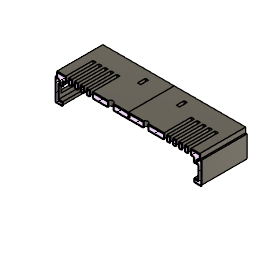
10.1 Screen Case Assembly (Autodesk Fusion 360 design; units mm, degrees)
part number: 2026-02-22-22-43-30-238
Autodesk Fusion 360 part; units mm, degrees
note: some values were not read from the file. Set by a fixed rule: which face or edge a step refers to.
(part 1 of 2)
sketch "Sketch1" plane through (0, 0, 0) normal (0, 0, 1) x (1, 0, 0)
  line L0 (117.5, -71.5) -> (-117.5, -71.5)
  line L1 (-117.5, -71.5) -> (-117.5, 71.5)
  line L2 (-117.5, 71.5) -> (117.5, 71.5)
  line L3 (117.5, 71.5) -> (117.5, -71.5)
  line L4 (117.5, -71.5) -> (-117.5, 71.5) construction
  line L5 (-117.5, -71.5) -> (117.5, 71.5) construction
  line L6 (-112.5, -66.5) -> (-112.5, 66.5)
  line L7 (-112.5, 66.5) -> (112.5, 66.5)
  line L8 (112.5, 66.5) -> (112.5, -66.5)
  line L9 (112.5, -66.5) -> (-112.5, -66.5)
  line L10 (122.5, -76.5) -> (-122.5, -76.5)
  line L11 (-122.5, -76.5) -> (-122.5, 76.5)
  line L12 (-122.5, 76.5) -> (122.5, 76.5)
  line L13 (122.5, 76.5) -> (122.5, -76.5)
  dimension "d1" = 235
  dimension "d2" = 143
  dimension "d3" = 5
  dimension "d4" = -5
  constraint horizontal L0
  constraint perpendicular L0 L1
  constraint parallel L0 L2
  constraint parallel L1 L3
  constraint coincident L4 origin
  constraint coincident L5 origin
  measures "d1" distance of L1.end L2.end
  measures "d2" distance of L0.end L1.end
extrude "Extrude1" add sketch "Sketch1" along normal blind 25 contours L0 L1 L2 L3 | L10 L11 L12 L13 makes body 1
ref_plane "WorkPlane1" through (0, 0, 12.5) normal (1, 0, 0) x (0, 1, 0)
sketch "Sketch2" plane through (0, 0, 0) normal (0, 0, -1) x (1, 0, 0)
  line L0 (112.5, 66.5) -> (112.5, -66.5)
  line L1 (112.5, -66.5) -> (-112.5, -66.5)
  line L2 (-112.5, -66.5) -> (-112.5, 66.5)
  line L3 (-112.5, 66.5) -> (112.5, 66.5)
  line L4 (-122.5, -76.5) -> (122.5, -76.5)
  line L5 (122.5, -76.5) -> (122.5, 76.5)
  line L6 (122.5, 76.5) -> (-122.5, 76.5)
  line L7 (-122.5, 76.5) -> (-122.5, -76.5)
sketch "Sketch3" plane through (0, 0, 25) normal (0, 0, 1) x (-1, 0, 0)
  line L0 (-112.5, -66.5) -> (-112.5, 66.5)
  line L1 (-112.5, 66.5) -> (112.5, 66.5)
  line L2 (112.5, 66.5) -> (112.5, -66.5)
  line L3 (112.5, -66.5) -> (-112.5, -66.5)
  line L4 (-122.5, -76.5) -> (122.5, -76.5)
  line L5 (122.5, -76.5) -> (122.5, 76.5)
  line L6 (122.5, 76.5) -> (-122.5, 76.5)
  line L7 (-122.5, 76.5) -> (-122.5, -76.5)
  line L8 (-112.5, 66.5) -> (112.5, 66.5)
  line L9 (-117.5, -71.5) -> (117.5, 71.5) construction
  line L10 (122.5, 76.5) -> (122.5, -76.5)
  line L11 (-112.5, -66.5) -> (-112.5, 66.5)
  line L12 (117.5, -71.5) -> (-117.5, 71.5) construction
  line L13 (117.5, -71.5) -> (-117.5, -71.5)
  line L14 (117.5, 71.5) -> (117.5, -71.5)
  line L15 (112.5, -66.5) -> (-112.5, -66.5)
  line L16 (-117.5, -71.5) -> (-117.5, 71.5)
  line L17 (-122.5, -76.5) -> (-122.5, 76.5)
  line L18 (112.5, 66.5) -> (112.5, -66.5)
  line L19 (-122.5, 76.5) -> (122.5, 76.5)
  line L20 (-117.5, 71.5) -> (117.5, 71.5)
  line L21 (122.5, -76.5) -> (-122.5, -76.5)
  dimension "d7" = 5
  dimension "d8" = -5
  dimension "d9" = 235
  dimension "d10" = 143
  constraint horizontal L13
  constraint perpendicular L13 L16
  constraint parallel L13 L20
  constraint parallel L14 L16
  constraint coincident origin L12
  constraint coincident origin L9
  measures "d9" distance of L12.end L9.end
  measures "d10" distance of L12.end L9.start
extrude "Extrude2" cut sketch "Sketch3" against normal blind 20 contours L13 L14 L16 L20 bodies 1
sketch "Sketch5" plane through (0, -71.5, 0) normal (0, 1, 0) x (-1, 0, 0)
  line L0 (117.5, 25) -> (-117.5, 25)
  line L1 (-117.5, 25) -> (-117.5, 5)
  line L2 (-117.5, 5) -> (117.5, 5)
  line L3 (117.5, 5) -> (117.5, 25)
sketch "Sketch6" plane through (0, 76.5, 0) normal (0, 1, 0) x (-1, 0, 0)
  line L0 (-122.5, 0) -> (122.5, 0)
  line L1 (122.5, 0) -> (122.5, 25)
  line L2 (122.5, 25) -> (-122.5, 25)
  line L3 (-122.5, 25) -> (-122.5, 0)
  line L4 (122.5, 25) -> (-122.5, 25)
  line L5 (-122.5, 25) -> (-122.5, 0)
  line L6 (-122.5, 0) -> (122.5, 0)
  line L7 (122.5, 0) -> (122.5, 25)
  line L8 (-117.5, 5) -> (117.5, 5)
  line L9 (117.5, 5) -> (117.5, 25)
  line L10 (117.5, 25) -> (-117.5, 25)
  line L11 (-117.5, 25) -> (-117.5, 5)
  line L12 (-117.5, 5) -> (-94.5, 5)
  line L13 (-94.5, 5) -> (-59, 5)
  line L14 (-59, 5) -> (-59, 12)
  line L15 (-59, 12) -> (-94.5, 12)
  line L16 (-94.5, 12) -> (-94.5, 5)
  dimension "d19" = 23
  dimension "d20" = 35.5
  dimension "d21" = 7
  constraint horizontal L4
  constraint vertical L5
  constraint horizontal L6
  constraint vertical L7
  constraint coincident L0.start L3.end
  constraint coincident L1.end L2.start
  constraint horizontal L8
  constraint vertical L9
  constraint horizontal L10
  constraint vertical L11
  constraint coincident L4 L9.end
  constraint horizontal L12
  constraint horizontal L13
  constraint vertical L14
  constraint horizontal L15
  constraint vertical L16
  measures "d19" distance of L8.start L12.end
  measures "d20" distance of L12.end L13.end
  measures "d21" distance of L12.end L15.end
extrude "Extrude3" cut sketch "Sketch6" against normal blind 8 contours L8 L13 L14 L15 L16 bodies 1
sketch "Sketch7" plane through (-117.5, 0, 0) normal (1, 0, 0) x (0, 1, 0)
  line L0 (71.5, 25) -> (-71.5, 25)
  line L1 (-71.5, 25) -> (-71.5, 5)
  line L2 (-71.5, 5) -> (71.5, 5)
  line L3 (71.5, 5) -> (71.5, 25)
  line L4 (71.5, 5) -> (44.8, 5)
  line L5 (50, 5) -> (14.4, 5)
  line L6 (14.4, 5) -> (14.4, 12)
  line L7 (14.4, 12) -> (50, 12)
  line L8 (50, 12) -> (50, 5)
  dimension "d24" = 26.7
  dimension "d25" = 35.6
  dimension "d26" = 7
  constraint coincident L2.end L3.start
  constraint perpendicular L3 L4
  constraint horizontal L5
  constraint vertical L6
  constraint horizontal L7
  constraint vertical L8
  constraint coincident L4 L5.start
  measures "d24" distance of L2.end L4.end
  measures "d25" distance of L5.start L5.end
  measures "d26" distance of L5.start L7.end
extrude "Extrude4" cut sketch "Sketch7" against normal blind 20 contours L2 L4 L5 L6 L7 L8 bodies 1
sketch "Sketch8" plane through (0, -76.5, 0) normal (0, -1, 0) x (1, 0, 0)
  line L0 (-122.5, 0) -> (122.5, 0)
  line L1 (122.5, 0) -> (122.5, 25)
  line L2 (122.5, 25) -> (-122.5, 25)
  line L3 (-122.5, 25) -> (-122.5, 0)
  line L4 (0, 0) -> (0, 30)
  constraint coincident L4.start origin
  constraint perpendicular L0 L4
sketch "Sketch9" plane through (0, 71.5, 0) normal (0, -1, 0) x (1, 0, 0)
  line L0 (117.5, 25) -> (-117.5, 25)
  line L1 (-117.5, 25) -> (-117.5, 5)
  line L2 (94.5, 5) -> (117.5, 5)
  line L3 (-117.5, 25) -> (117.5, 25)
  line L4 (117.5, 25) -> (117.5, 5)
  line L5 (117.5, 5) -> (-117.5, 5)
  line L6 (-117.5, 5) -> (-117.5, 25)
  line L7 (-117.5, 10.0628) -> (117.5, 10.0628)
  line L8 (117.5, 10.0628) -> (117.5, 15)
  line L9 (117.5, 15) -> (-117.5, 15)
  line L10 (-117.5, 15) -> (-117.5, 10.0628)
  line L11 (59, 5) -> (59, 12)
  line L12 (59, 12) -> (94.5, 12)
  line L13 (94.5, 12) -> (94.5, 5)
  line L14 (117.5, 5) -> (117.5, 25)
  line L15 (-117.5, 5) -> (59, 5)
  constraint horizontal L3
  constraint vertical L4
  constraint horizontal L5
  constraint vertical L6
  constraint coincident L2.end L4.end
  constraint coincident L0.end L1.start
  constraint horizontal L7
  constraint vertical L8
  constraint horizontal L9
  constraint vertical L10
  constraint midpoint L4 L8.end
  constraint coincident L6 L7.start
sketch "Sketch10" plane through (0, 0, 5) normal (0, 0, 1) x (-1, 0, 0)
  line L0 (-59, -71.5) -> (117.5, -71.5)
  line L1 (117.5, -71.5) -> (117.5, -50)
  line L2 (117.5, -50) -> (122.5, -50)
  line L3 (122.5, -50) -> (122.5, -14.4)
  line L4 (122.5, -14.4) -> (117.5, -14.4)
  line L5 (117.5, -14.4) -> (117.5, 71.5)
  line L6 (117.5, 71.5) -> (-117.5, 71.5)
  line L7 (-117.5, 71.5) -> (-117.5, -71.5)
  line L8 (-117.5, -71.5) -> (-94.5, -71.5)
  line L9 (-94.5, -71.5) -> (-94.5, -76.5)
  line L10 (-94.5, -76.5) -> (-59, -76.5)
  line L11 (-59, -76.5) -> (-59, -71.5)
  line L12 (-112.5, 66.5) -> (112.5, 66.5)
  line L13 (112.5, 66.5) -> (112.5, -66.5)
  line L14 (112.5, -66.5) -> (-112.5, -66.5)
  line L15 (-112.5, -66.5) -> (-112.5, 66.5)
  line L16 (117.5, -14.4) -> (122.5, -14.4)
  line L17 (122.5, -14.4) -> (122.5, -50)
  line L18 (122.5, -50) -> (117.5, -50)
  line L19 (117.5, -50) -> (117.5, -14.4)
  line L20 (117.5, -32.2) -> (122.5, -32.2)
  line L21 (120, -14.4) -> (120, -32.2)
  line L22 (120.4, -23.4) -> (119.6, -23.4)
  line L23 (119.6, -23.4) -> (119.6, -22.6)
  line L24 (119.6, -22.6) -> (120.4, -22.6)
  line L25 (120.4, -22.6) -> (120.4, -23.4)
  line L26 (120.4, -23.4) -> (119.6, -22.6) construction
  line L27 (119.6, -23.4) -> (120.4, -22.6) construction
  line L28 (120.4, -27.6) -> (119.6, -27.6)
  line L29 (119.6, -27.6) -> (119.6, -28.4)
  line L30 (119.6, -28.4) -> (120.4, -28.4)
  line L31 (120.4, -28.4) -> (120.4, -27.6)
  line L32 (120.4, -27.6) -> (119.6, -28.4) construction
  line L33 (119.6, -27.6) -> (120.4, -28.4) construction
  line L34 (120.4, -36) -> (120.4, -36.8)
  line L35 (120.4, -36.8) -> (119.6, -36.8)
  line L36 (119.6, -36.8) -> (119.6, -36)
  line L37 (119.6, -36) -> (120.4, -36)
  line L38 (120.4, -41.8) -> (120.4, -41)
  line L39 (119.6, -41.8) -> (120.4, -41.8)
  line L40 (120.4, -41) -> (119.6, -41)
  line L41 (119.6, -41) -> (119.6, -41.8)
  line L42 (120.4, -17.6) -> (119.6, -17.6)
  line L43 (119.6, -17.6) -> (119.6, -18.4)
  line L44 (119.6, -18.4) -> (120.4, -18.4)
  line L45 (120.4, -18.4) -> (120.4, -17.6)
  line L46 (120.4, -17.6) -> (119.6, -18.4) construction
  line L47 (119.6, -17.6) -> (120.4, -18.4) construction
  line L48 (119.6, -46.8) -> (119.6, -46)
  line L49 (120.4, -46.8) -> (119.6, -46.8)
  line L50 (120.4, -46) -> (120.4, -46.8)
  line L51 (119.6, -46) -> (120.4, -46)
  line L52 (119.6, -31.8) -> (120.4, -31.8)
  line L53 (120.4, -31.8) -> (120.4, -32.6)
  line L54 (120.4, -32.6) -> (119.6, -32.6)
  line L55 (119.6, -32.6) -> (119.6, -31.8)
  line L56 (119.6, -31.8) -> (120.4, -32.6) construction
  line L57 (120.4, -31.8) -> (119.6, -32.6) construction
  point P0 (120, -23)
  point P1 (120, -28)
  point P2 (120, -18)
  point P3 (120, -46.4)
  point P4 (120, -32.2)
  dimension "d32" = 0.8
  dimension "d33" = 0.8
  dimension "d34" = 0.8
  dimension "d35" = 0.8
  dimension "d38" = 0.8
  dimension "d39" = 0.8
  dimension "d56" = 0.8
  dimension "d57" = 0.8
  constraint horizontal L16
  constraint vertical L17
  constraint horizontal L18
  constraint vertical L19
  constraint coincident L2.end L3.start
  constraint coincident L4.end L5.start
  constraint midpoint L19 L20.start
  constraint midpoint L3 L20.end
  constraint midpoint L4 L21.start
  constraint midpoint L20 P4
  constraint horizontal L22
  constraint perpendicular L22 L23
  constraint parallel L22 L24
  constraint parallel L23 L25
  constraint coincident L26 P0
  constraint coincident L27 P0
  constraint coincident L21 P0
  constraint horizontal L28
  constraint perpendicular L28 L29
  constraint parallel L28 L30
  constraint parallel L29 L31
  constraint coincident L32 P1
  constraint coincident L33 P1
  constraint coincident L21 P1
  constraint symmetric L20 L22.start L38.end
  constraint symmetric L20 L22.end L40.end
  constraint symmetric L20 L23.end L39.start
  constraint symmetric L20 L24.end L38.start
  constraint symmetric L20 L28.start L34.end
  constraint symmetric L20 L28.end L35.end
  constraint symmetric L20 L29.end L36.end
  constraint symmetric L20 L30.end L34.start
  constraint horizontal L42
  constraint perpendicular L42 L43
  constraint parallel L42 L44
  constraint parallel L43 L45
  constraint coincident L46 P2
  constraint coincident L47 P2
  constraint coincident L21 P2
  constraint symmetric L20 L42.start L49.start
  constraint symmetric L20 L42.end L48.start
  constraint symmetric L20 L43.end L48.end
  constraint symmetric L20 L44.end L50.start
  constraint symmetric L20 P2 P3
  constraint horizontal L52
  constraint perpendicular L52 L53
  constraint parallel L52 L54
  constraint parallel L53 L55
  constraint coincident L56 P4
  constraint coincident L57 P4
  constraint coincident P4 L21.end
  measures "d32" distance of L23.end L24.end
  measures "d33" distance of L22.end L23.end
  measures "d34" distance of L29.end L30.end
  measures "d35" distance of L28.end L29.end
  measures "d38" distance of L43.end L44.end
  measures "d39" distance of L42.end L43.end
  measures "d56" distance of L53.end L54.end
  measures "d57" distance of L52.end L53.end
sketch "Sketch11" plane through (0, 0, 5) normal (0, 0, 1) x (-1, 0, 0)
  line L0 (-59, -71.5) -> (117.5, -71.5)
  line L1 (117.5, -71.5) -> (117.5, -50)
  line L2 (117.5, -50) -> (122.5, -50)
  line L3 (122.5, -50) -> (122.5, -14.4)
  line L4 (122.5, -14.4) -> (117.5, -14.4)
  line L5 (117.5, -14.4) -> (117.5, 71.5)
  line L6 (117.5, 71.5) -> (-117.5, 71.5)
  line L7 (-117.5, 71.5) -> (-117.5, -71.5)
  line L8 (-117.5, -71.5) -> (-94.5, -71.5)
  line L9 (-94.5, -71.5) -> (-94.5, -76.5)
  line L10 (-94.5, -76.5) -> (-59, -76.5)
  line L11 (-59, -76.5) -> (-59, -71.5)
  line L12 (-112.5, 66.5) -> (112.5, 66.5)
  line L13 (112.5, 66.5) -> (112.5, -66.5)
  line L14 (112.5, -66.5) -> (-112.5, -66.5)
  line L15 (-112.5, -66.5) -> (-112.5, 66.5)
  line L16 (-59, -76.5) -> (-94.5, -76.5)
  line L17 (-94.5, -76.5) -> (-94.5, -71.5)
  line L18 (-94.5, -71.5) -> (-59, -71.5)
  line L19 (-59, -71.5) -> (-59, -76.5)
  line L20 (-77.15, -73.6) -> (-76.35, -73.6)
  line L21 (-76.35, -73.6) -> (-76.35, -74.4)
  line L22 (-76.35, -74.4) -> (-77.15, -74.4)
  line L23 (-77.15, -74.4) -> (-77.15, -73.6)
  line L24 (-77.15, -73.6) -> (-76.35, -74.4) construction
  line L25 (-76.35, -73.6) -> (-77.15, -74.4) construction
  line L26 (-61.4, -73.6) -> (-60.6, -73.6)
  line L27 (-60.6, -73.6) -> (-60.6, -74.4)
  line L28 (-60.6, -74.4) -> (-61.4, -74.4)
  line L29 (-61.4, -74.4) -> (-61.4, -73.6)
  line L30 (-61.4, -73.6) -> (-60.6, -74.4) construction
  line L31 (-60.6, -73.6) -> (-61.4, -74.4) construction
  line L32 (-64.4, -73.6) -> (-63.6, -73.6)
  line L33 (-63.6, -73.6) -> (-63.6, -74.4)
  line L34 (-63.6, -74.4) -> (-64.4, -74.4)
  line L35 (-64.4, -74.4) -> (-64.4, -73.6)
  line L36 (-64.4, -73.6) -> (-63.6, -74.4) construction
  line L37 (-63.6, -73.6) -> (-64.4, -74.4) construction
  line L38 (-66.6, -73.6) -> (-67.4, -73.6)
  line L39 (-67.4, -73.6) -> (-67.4, -74.4)
  line L40 (-67.4, -74.4) -> (-66.6, -74.4)
  line L41 (-66.6, -74.4) -> (-66.6, -73.6)
  line L42 (-66.6, -73.6) -> (-67.4, -74.4) construction
  line L43 (-67.4, -73.6) -> (-66.6, -74.4) construction
  line L44 (-71.4, -73.6) -> (-70.6, -73.6)
  line L45 (-70.6, -73.6) -> (-70.6, -74.4)
  line L46 (-70.6, -74.4) -> (-71.4, -74.4)
  line L47 (-71.4, -74.4) -> (-71.4, -73.6)
  line L48 (-71.4, -73.6) -> (-70.6, -74.4) construction
  line L49 (-70.6, -73.6) -> (-71.4, -74.4) construction
  line L50 (-74.4, -73.6) -> (-73.6, -73.6)
  line L51 (-73.6, -73.6) -> (-73.6, -74.4)
  line L52 (-73.6, -74.4) -> (-74.4, -74.4)
  line L53 (-74.4, -74.4) -> (-74.4, -73.6)
  line L54 (-74.4, -73.6) -> (-73.6, -74.4) construction
  line L55 (-73.6, -73.6) -> (-74.4, -74.4) construction
  line L56 (-79.9, -74.4) -> (-79.1, -74.4)
  line L57 (-86.1, -74.4) -> (-86.9, -74.4)
  line L58 (-82.1, -73.6) -> (-82.9, -74.4) construction
  line L59 (-82.9, -73.6) -> (-82.1, -74.4) construction
  line L60 (-86.1, -73.6) -> (-86.9, -74.4) construction
  line L61 (-79.1, -73.6) -> (-79.9, -73.6)
  line L62 (-79.1, -73.6) -> (-79.9, -74.4) construction
  line L63 (-92.9, -73.6) -> (-92.9, -74.4)
  line L64 (-86.1, -73.6) -> (-86.1, -74.4)
  line L65 (-89.9, -73.6) -> (-89.1, -74.4) construction
  line L66 (-82.9, -74.4) -> (-82.1, -74.4)
  line L67 (-92.1, -73.6) -> (-92.9, -74.4) construction
  line L68 (-82.1, -73.6) -> (-82.9, -73.6)
  line L69 (-89.9, -73.6) -> (-89.9, -74.4)
  line L70 (-92.1, -73.6) -> (-92.9, -73.6)
  line L71 (-86.9, -74.4) -> (-86.9, -73.6)
  line L72 (-86.9, -73.6) -> (-86.1, -74.4) construction
  line L73 (-86.9, -73.6) -> (-86.1, -73.6)
  line L74 (-92.9, -73.6) -> (-92.1, -74.4) construction
  line L75 (-82.9, -73.6) -> (-82.9, -74.4)
  line L76 (-92.1, -74.4) -> (-92.1, -73.6)
  line L77 (-89.1, -73.6) -> (-89.9, -74.4) construction
  line L78 (-89.9, -74.4) -> (-89.1, -74.4)
  line L79 (-79.9, -73.6) -> (-79.1, -74.4) construction
  line L80 (-89.1, -74.4) -> (-89.1, -73.6)
  line L81 (-89.1, -73.6) -> (-89.9, -73.6)
  line L82 (-92.9, -74.4) -> (-92.1, -74.4)
  line L83 (-82.1, -74.4) -> (-82.1, -73.6)
  line L84 (-79.1, -74.4) -> (-79.1, -73.6)
  line L85 (-79.9, -73.6) -> (-79.9, -74.4)
  point P0 (-76.75, -74)
  point P1 (-61, -74)
  point P2 (-64, -74)
  point P3 (-67, -74)
  point P4 (-71, -74)
  point P5 (-74, -74)
  point P6 (-89.5, -74)
  point P7 (-79.5, -74)
  point P8 (-86.5, -74)
  point P9 (-82.5, -74)
  point P10 (-92.5, -74)
  dimension "d42" = 0.8
  dimension "d43" = 0.8
  dimension "d44" = 0.8
  dimension "d45" = 0.8
  dimension "d46" = 0.8
  dimension "d47" = 0.8
  dimension "d48" = 0.8
  dimension "d49" = 0.8
  dimension "d50" = 0.8
  dimension "d51" = 0.8
  dimension "d52" = 0.8
  dimension "d53" = 0.8
  constraint horizontal L16
  constraint vertical L17
  constraint horizontal L18
  constraint vertical L19
  constraint coincident L8.end L9.start
  constraint coincident L10.end L11.start
  constraint horizontal L20
  constraint perpendicular L20 L21
  constraint parallel L20 L22
  constraint parallel L21 L23
  constraint coincident L24 P0
  constraint coincident L25 P0
  constraint horizontal L26
  constraint perpendicular L26 L27
  constraint parallel L26 L28
  constraint parallel L27 L29
  constraint coincident L30 P1
  constraint coincident L31 P1
  constraint horizontal L32
  constraint perpendicular L32 L33
  constraint parallel L32 L34
  constraint parallel L33 L35
  constraint coincident L36 P2
  constraint coincident L37 P2
  constraint horizontal L38
  constraint perpendicular L38 L39
  constraint parallel L38 L40
  constraint parallel L39 L41
  constraint coincident L42 P3
  constraint coincident L43 P3
  constraint horizontal L44
  constraint perpendicular L44 L45
  constraint parallel L44 L46
  constraint parallel L45 L47
  constraint coincident L48 P4
  constraint coincident L49 P4
  constraint horizontal L50
  constraint perpendicular L50 L51
  constraint parallel L50 L52
  constraint parallel L51 L53
  constraint coincident L54 P5
  constraint coincident L55 P5
  measures "d42" distance of L21.end L22.end
  measures "d43" distance of L20.end L21.end
  measures "d44" distance of L27.end L28.end
  measures "d45" distance of L26.end L27.end
  measures "d46" distance of L33.end L34.end
  measures "d47" distance of L32.end L33.end
  measures "d48" distance of L39.end L40.end
  measures "d49" distance of L38.end L39.end
  measures "d50" distance of L45.end L46.end
  measures "d51" distance of L44.end L45.end
  measures "d52" distance of L51.end L52.end
  measures "d53" distance of L50.end L51.end
split "Split4" by plane through (0, 0, 0) normal (0, 1, 0) bodies 1 makes body 2 at (-62, 76.5, 12.3333)
move_body "Move5" bodies 1 to x (1, 0, 0) y (0, 1, 0) z (0, 0, 1) at (0, -2.5, 0)
sketch "Sketch12" plane through (0, 0, 0) normal (0, -1, 0) x (1, 0, 0)
  line L0 (-112.5, 0) -> (-112.5, 5)
  line L1 (-112.5, 5) -> (-117.5, 5)
  line L2 (-117.5, 5) -> (-117.5, 25)
  line L3 (-117.5, 25) -> (-122.5, 25)
  line L4 (-122.5, 25) -> (-122.5, 0)
  line L5 (-122.5, 0) -> (-112.5, 0)
  line L6 (-122.5, 25) -> (-122.5, 0)
  line L7 (-114.5, 0) -> (-112.5, 2)
  line L8 (-114.5, 0) -> (-122.5, 0)
  line L9 (-112.5, 2) -> (-112.5, 5)
  line L10 (-117.5, 5) -> (-112.5, 5)
  line L11 (-122.5, 25) -> (-117.5, 25)
  line L12 (-117.5, 25) -> (-117.5, 5)
  line L13 (0, 1.75) -> (0, 22.5)
  line L14 (117.5, 25) -> (122.5, 25)
  line L15 (112.5, 2) -> (112.5, 5)
  line L16 (117.5, 5) -> (117.5, 25)
  line L17 (114.5, 0) -> (112.5, 2)
  line L18 (112.5, 5) -> (117.5, 5)
  line L19 (117.5, 25) -> (117.5, 5)
  line L20 (122.5, 25) -> (122.5, 0)
  line L21 (117.5, 5) -> (112.5, 5)
  line L22 (114.5, 0) -> (112.5, 2)
  line L23 (112.5, 2) -> (112.5, 5)
  line L24 (122.5, 25) -> (122.5, 0)
  line L25 (122.5, 0) -> (114.5, 0)
  line L26 (122.5, 25) -> (117.5, 25)
  line L27 (114.5, 0) -> (122.5, 0)
  constraint coincident L3.end L4.start
  constraint coincident L4.end L5.start
  constraint coincident L0.start L7.start
  constraint coincident L0.start L7.end
  constraint coincident L0.end L1.start
  constraint coincident L1.end L2.start
  constraint coincident L2.end L3.start
  constraint symmetric L0.end L13 L15.end
  constraint symmetric L1.end L13 L16.start
  constraint symmetric L2.end L13 L14.start
  constraint symmetric L3.end L13 L14.end
  constraint symmetric L4.end L13 L20.end
  constraint symmetric L7.start L13 L17.start
  constraint symmetric L7.end L13 L15.start
extrude "Extrude10" add sketch "Sketch12" along normal up to surface (2.5 mm away) contours L0 L1 L2 L3 L4 L5 L6 L7 L8 L9 L10 L11 L12 | L14 L15 L16 L17 L18 L19 L20 L21 L22 L23 L24 L25 L26 L27 bodies 1 2
ref_plane "WorkPlane3" through (0, -1.25, 12.5) normal (0, -1, 0) x (1, 0, 0)
sketch "Sketch13" plane through (0, 0, 25) normal (0, 0, 1) x (-1, 0, 0)
  line L0 (117.5, 74) -> (117.5, -71.5)
  line L1 (117.5, -71.5) -> (-117.5, -71.5)
  line L2 (-117.5, -71.5) -> (-117.5, 74)
  line L3 (-117.5, 74) -> (117.5, 74)
  line L4 (122.5, -76.5) -> (122.5, 79)
  line L5 (122.5, 79) -> (-122.5, 79)
  line L6 (-122.5, 79) -> (-122.5, -76.5)
  line L7 (-122.5, -76.5) -> (122.5, -76.5)
  line L8 (-122.5, 79) -> (122.5, 79)
  line L9 (122.5, 79) -> (122.5, -76.5)
  line L10 (122.5, -76.5) -> (-122.5, -76.5)
  line L11 (-122.5, -76.5) -> (-122.5, 79)
  line L12 (-117.5, 74) -> (117.5, 74)
  line L13 (117.5, 74) -> (117.5, -71.5)
  line L14 (117.5, -71.5) -> (-117.5, -71.5)
  line L15 (-117.5, -71.5) -> (-117.5, 74)
  constraint horizontal L8
  constraint vertical L9
  constraint horizontal L10
  constraint vertical L11
  constraint coincident L4.start L7.end
  constraint coincident L5.end L6.start
  constraint horizontal L12
  constraint vertical L13
  constraint horizontal L14
  constraint vertical L15
  constraint coincident L0.end L1.start
  constraint coincident L2.end L3.start
extrude "Extrude11" add sketch "Sketch13" along normal blind 11.5 bodies 1
extrude "Extrude12" add 1 faces at (-113.1667, 0, 0.6667) along direction (0, -1, 0) blind 3 on bodies 1 bodies 1
extrude "Extrude13" add 1 faces at (113.1667, 0, 0.6667) along direction (0, -1, 0) blind 3 on bodies 1 bodies 1
sketch "Sketch14" plane through (-117.5, 0, 0) normal (1, 0, 0) x (0, 1, 0)
  line L0 (-74, 5) -> (14.4, 5)
  line L1 (14.4, 5) -> (14.4, 12)
  line L2 (14.4, 12) -> (50, 12)
  line L3 (50, 12) -> (50, 5)
  line L4 (50, 5) -> (71.5, 5)
  line L5 (71.5, 5) -> (71.5, 36.5)
  line L6 (71.5, 36.5) -> (-74, 36.5)
  line L7 (-74, 36.5) -> (-74, 5)
  line L8 (30, 12) -> (0, 12)
  line L9 (0, 12) -> (0, 22)
  line L10 (0, 22) -> (30, 22)
  line L11 (30, 22) -> (30, 12)
  dimension "d70" = 30
  constraint horizontal L8
  constraint vertical L9
  constraint horizontal L10
  constraint vertical L11
  constraint coincident L2 L8.start
  measures "d70" distance of L8.start L8.end
extrude "Extrude14" add 1 faces at (-119.1667, 50, 9.6667) along direction (0, -1, 0) blind 36 on bodies 1 bodies 1
extrude "Extrude15" cut sketch "Sketch14" against normal blind 15 contours L2 L8 L9 L10 L11 bodies 1
sketch "Sketch15" plane through (0, 71.5, 0) normal (0, -1, 0) x (1, 0, 0)
  line L0 (59, 5) -> (59, 12)
  line L1 (59, 12) -> (94.5, 12)
  line L2 (94.5, 12) -> (94.5, 5)
  line L3 (94.5, 5) -> (117.5, 5)
  line L4 (117.5, 5) -> (117.5, 36.5)
  line L5 (117.5, 36.5) -> (-117.5, 36.5)
  line L6 (-117.5, 36.5) -> (-117.5, 5)
  line L7 (-117.5, 5) -> (59, 5)
  line L8 (59, 12) -> (59, 25.5)
  line L9 (85, 12) -> (35, 12)
  line L10 (35, 12) -> (35, 24)
  line L11 (35, 24) -> (85, 24)
  line L12 (85, 24) -> (85, 12)
  dimension "d75" = 13.5
  constraint coincident L0.end L1.start
  constraint perpendicular L1 L8
  constraint horizontal L9
  constraint vertical L10
  constraint horizontal L11
  constraint vertical L12
  constraint coincident L1 L9.start
  measures "d75" distance of L0.end L8.end
extrude "Extrude16" add 1 faces at (94.5, 73.1667, 7.3333) along direction (-1, 0, 0) blind 36 on bodies 1 bodies 1
extrude "Extrude17" cut sketch "Sketch15" against normal blind 12 contours L1 L8 L9 L11 L12 | L8 L9 L10 L11 bodies 1
extrude "Extrude18" add 1 faces at (112.5, 21.3333, 1.6667) along direction (-1, 0, 0) blind 2 on bodies 1 bodies 1
extrude "Extrude19" add 1 faces at (36.1667, -69, 1.6667) along direction (0, 1, 0) blind 2 on bodies 1 bodies 1
extrude "Extrude20" add 1 faces at (-38.1667, 66.5, 1.6667) along direction (0, -1, 0) blind 2 on bodies 1 bodies 1
extrude "Extrude21" add 1 faces at (-112.5, 20.6667, 3.3333) along direction (1, 0, 0) blind 2 on bodies 1 bodies 1
ref_plane "WorkPlane4" through (0, -1.25, 18.25) normal (-1, 0, 0) x (0, -1, 0)
sketch "Sketch16" plane through (-117.5, 0, 0) normal (1, 0, 0) x (0, 1, 0)
  line L0 (0, 12) -> (0, 22)
  line L1 (0, 22) -> (30, 22)
  line L2 (30, 22) -> (30, 12)
  line L3 (30, 12) -> (0, 12)
  line L4 (-74, 5) -> (71.5, 5)
  line L5 (71.5, 36.5) -> (-74, 36.5)
  line L6 (-74, 36.5) -> (-74, 5)
  line L7 (-74, 5) -> (71.629, 5)
  line L8 (71.629, 5) -> (71.629, 12.4)
  line L9 (71.629, 12.4) -> (-74, 12.4)
  line L10 (-74, 12.4) -> (-74, 5)
  line L11 (71.629, 12.4) -> (61.629, 12.4)
  line L12 (71.629, 17.4) -> (71.629, 12.4)
  line L13 (71.629, 12.4) -> (71.629, 12.9)
  line L14 (71.5, 5) -> (71.629, 12.9)
  line L15 (71.629, 12.9) -> (51.629, 12.9)
  line L16 (51.629, 12.9) -> (51.629, 18.9)
  line L17 (51.629, 18.9) -> (71.629, 18.9)
  line L18 (71.629, 18.9) -> (71.629, 12.9)
  dimension "d88" = 7.4
  dimension "d89" = 10
  dimension "d90" = 5
  dimension "d105" = 0.5
  dimension "d106" = 20
  dimension "d107" = 6
  constraint horizontal L7
  constraint vertical L8
  constraint horizontal L9
  constraint vertical L10
  constraint coincident L4.start L6.end
  constraint horizontal L11
  constraint vertical L12
  constraint vertical L13
  constraint coincident L4.end L14.start
  constraint horizontal L15
  constraint vertical L16
  constraint horizontal L17
  constraint vertical L18
  measures "d88" distance of L4.start L9.end
  measures "d89" distance of L8.end L11.end
  measures "d90" distance of L8.end L12.start
  measures "d105" distance of L8.end L13.end
  measures "d106" distance of L13.end L15.end
  measures "d107" distance of L13.end L17.end
extrude "Extrude26" add sketch "Sketch16" along normal blind 7 contours L12 L15 L16 L17 L18 bodies 1
sketch "Sketch18" plane through (-110.5, 0, 0) normal (1, 0, 0) x (0, 1, 0)
  line L0 (71.5, 12.9) -> (71.5, 18.9)
  line L1 (71.5, 18.9) -> (51.629, 18.9)
  line L2 (51.629, 18.9) -> (51.629, 12.9)
  line L3 (51.629, 12.9) -> (71.5, 12.9)
  line L4 (64.5, 5) -> (64.5, 18.9)
  line L5 (64.5, 18.9) -> (71.5, 18.9)
  line L6 (71.5, 18.9) -> (71.5, 12.9)
  line L7 (71.5, 12.9) -> (64.5, 12.9)
  line L8 (64.5, 12.9) -> (64.5, 18.9)
  constraint coincident L1 L4.end
  constraint perpendicular L1 L4
  constraint horizontal L5
  constraint vertical L6
  constraint horizontal L7
  constraint vertical L8
  constraint coincident L0.start L3.end
extrude "Extrude27" add sketch "Sketch18" along normal blind 13 contours L0 L1 L3 L4 L5 L6 L7 L8 bodies 1
mirror "Mirror3" about plane through (0, -1.25, 12.5) normal (0, -1, 0) of "Extrude26", "Extrude27"
mirror "Mirror4" about plane through (0, -1.25, 18.25) normal (-1, 0, 0) of "Extrude26", "Extrude27", "Mirror3"
split "Split6" by plane through (0, -1.25, 18.25) normal (-1, 0, 0) bodies 1 makes body 3 at (-122.5, -52.6667, 19.5)
extrude "Extrude29" cut 1 faces at (-108.5, 69.1667, 12.9) along direction (0, 0, 1) blind 1 on bodies 3 bodies 3
extrude "Extrude30" add 1 faces at (-108.5, 69.1667, 18.9) along direction (0, 0, 1) blind 1 on bodies 3 bodies 3
sketch "Sketch19" plane through (-117.5, 0, 0) normal (1, 0, 0) x (0, 1, 0)
  line L0 (51.629, 13.9) -> (51.629, 19.9)
  line L1 (51.629, 19.9) -> (71.5, 19.9)
  line L2 (71.5, 19.9) -> (71.5, 36.5)
  line L3 (71.5, 36.5) -> (-74, 36.5)
  line L4 (-74, 36.5) -> (-74, 18.9)
  line L5 (-74, 18.9) -> (-54.129, 18.9)
  line L6 (-54.129, 18.9) -> (-54.129, 12.9)
  line L7 (-54.129, 12.9) -> (-74, 12.9)
  line L8 (-74, 12.9) -> (-74, 5)
  line L9 (-74, 5) -> (71.5, 5)
  line L10 (71.5, 5) -> (71.5, 13.9)
  line L11 (71.5, 13.9) -> (51.629, 13.9)
  line L12 (0, 12) -> (0, 22)
  line L13 (0, 22) -> (30, 22)
  line L14 (30, 22) -> (30, 12)
  line L15 (30, 12) -> (0, 12)
  line L16 (0, 22) -> (41.3847, 22)
  line L17 (41.3847, 22) -> (41.3847, 11.8033)
  line L18 (41.3847, 11.8033) -> (0, 11.8033)
  line L19 (0, 11.8033) -> (0, 22)
  line L20 (0, 11.8033) -> (41.3847, 11.8033)
  line L21 (41.3847, 11.8033) -> (41.3847, 26.3373)
  line L22 (41.3847, 26.3373) -> (0, 26.3373)
  line L23 (0, 26.3373) -> (0, 11.8033)
  constraint horizontal L16
  constraint vertical L17
  constraint horizontal L18
  constraint vertical L19
  constraint coincident L12.end L13.start
  constraint horizontal L20
  constraint vertical L21
  constraint horizontal L22
  constraint vertical L23
extrude "Extrude31" cut sketch "Sketch19" against normal blind 5 contours L14 L15 L16 L17 L18 L19 L20 L21 L23 | L13 L16 L21 L22 L23 bodies 3
sketch "Sketch20" plane through (0, 0, 11.8033) normal (0, 0, 1) x (-1, 0, 0)
  line L0 (117.5, 0) -> (117.5, -41.3847)
  line L1 (117.5, -41.3847) -> (122.5, -41.3847)
  line L2 (122.5, -41.3847) -> (122.5, 0)
  line L3 (122.5, 0) -> (117.5, 0)
  line L4 (122.5, -41.3847) -> (117.5, -41.3847)
  line L5 (117.5, -41.3847) -> (117.5, 0)
  line L6 (117.5, 0) -> (122.5, 0)
  line L7 (122.5, 0) -> (122.5, -41.3847)
  line L8 (120, -41.3847) -> (120, 0)
  line L9 (117.5, -20.6924) -> (123, -20.6924)
  line L10 (122.5, -19.6924) -> (117.5, -19.6924)
  line L11 (117.5, -19.6924) -> (117.5, -21.6924)
  line L12 (117.5, -21.6924) -> (122.5, -21.6924)
  line L13 (122.5, -21.6924) -> (122.5, -19.6924)
  line L14 (122.5, -19.6924) -> (117.5, -21.6924) construction
  line L15 (117.5, -19.6924) -> (122.5, -21.6924) construction
  point P0 (120, -20.6924)
  dimension "d124" = 2
  constraint horizontal L4
  constraint vertical L5
  constraint horizontal L6
  constraint vertical L7
  constraint coincident L0.start L3.end
  constraint coincident L1.end L2.start
  constraint midpoint L4 L8.start
  constraint midpoint L3 L8.end
  constraint midpoint L5 L9.start
  constraint perpendicular L7 L9
  constraint horizontal L10
  constraint perpendicular L10 L11
  constraint parallel L10 L12
  constraint parallel L11 L13
  constraint coincident L14 P0
  constraint coincident L15 P0
  constraint midpoint L8 P0
  measures "d124" distance of L10.end L11.end
extrude "Extrude32" add sketch "Sketch20" along normal up to surface (14.534 mm away) contours L0 L5 L8 L9 L10 L11 | L0 L5 L8 L9 L11 L12 | L2 L7 L8 L9 L10 L13 | L2 L7 L8 L9 L12 L13 bodies 3
sketch "Sketch21" plane through (0, 76.5, 0) normal (0, 1, 0) x (-1, 0, 0)
  line L0 (0, 0) -> (0, 36.5)
  line L1 (0, 36.5) -> (-122.5, 36.5)
  line L2 (-122.5, 36.5) -> (-122.5, 0)
  line L3 (-122.5, 0) -> (0, 0)
  line L4 (-35, 24) -> (-35, 12)
  line L5 (-35, 12) -> (-85, 12)
  line L6 (-85, 12) -> (-85, 24)
  line L7 (-85, 24) -> (-35, 24)
  line L8 (-85, 12) -> (-30, 12)
  line L9 (-30, 12) -> (-30, 28)
  line L10 (-30, 28) -> (-85, 28)
  line L11 (-85, 28) -> (-85, 12)
  constraint horizontal L8
  constraint vertical L9
  constraint horizontal L10
  constraint vertical L11
  constraint coincident L5.end L6.start
extrude "Extrude33" cut sketch "Sketch21" against normal blind 13 contours L4 L7 L8 L9 L10 L11 bodies 1
sketch "Sketch22" plane through (0, 0, 0) normal (-1, 0, 0) x (0, -1, 0)
  line L0 (-76.5, 36.5) -> (-76.5, 0)
  line L1 (-76.5, 0) -> (-64.5, 0)
  line L2 (-64.5, 0) -> (-64.5, 5)
  line L3 (-64.5, 5) -> (-71.5, 5)
  line L4 (-71.5, 5) -> (-71.5, 36.5)
  line L5 (-71.5, 36.5) -> (-76.5, 36.5)
  line L6 (-75.25, 35.25) -> (-75.25, 1.25)
  line L7 (-75.25, 1.25) -> (-65.75, 1.25)
  line L8 (-65.75, 1.25) -> (-65.75, 3.75)
  line L9 (-65.75, 3.75) -> (-72.75, 3.75)
  line L10 (-72.75, 3.75) -> (-72.75, 35.25)
  line L11 (-72.75, 35.25) -> (-75.25, 35.25)
  dimension "d129" = -1.25
extrude "Extrude34" add sketch "Sketch22" along normal blind 8 contours L6 L7 L8 L9 L10 L11 bodies 1
mirror "Mirror5" about plane through (0, -1.25, 12.5) normal (0, -1, 0) of 7 faces at (-2.6667, 72.75, 14.25) (-8, 74.4167, 13.4167) (-5.3333, 68.0833, 3.75) (-2.6667, 65.75, 2.0833) (-2.6667, 73.5833, 35.25) (-2.6667, 75.25, 23.9167) (-2.6667, 72.0833, 1.25) on bodies 1
sketch "Sketch23" plane through (0, 0, 0) normal (1, 0, 0) x (0, 1, 0)
  line L0 (76.5, 0) -> (76.5, 36.5)
  line L1 (76.5, 36.5) -> (71.5, 36.5)
  line L2 (71.5, 36.5) -> (71.5, 5)
  line L3 (71.5, 5) -> (64.5, 5)
  line L4 (64.5, 5) -> (64.5, 0)
  line L5 (64.5, 0) -> (76.5, 0)
  line L6 (72.75, 35.25) -> (72.75, 3.75)
  line L7 (72.75, 3.75) -> (65.75, 3.75)
  line L8 (65.75, 3.75) -> (65.75, 1.25)
  line L9 (65.75, 1.25) -> (75.25, 1.25)
  line L10 (75.25, 1.25) -> (75.25, 35.25)
  line L11 (75.25, 35.25) -> (72.75, 35.25)
  dimension "d134" = -1.25
extrude "Extrude35" cut sketch "Sketch23" against normal up to surface (8 mm away) contours L6 L7 L8 L9 L10 L11 bodies 3
mirror "Mirror6" about plane through (0, -1.25, 12.5) normal (0, -1, 0) of "Extrude35"
sketch "Sketch24" plane through (0, 0, 36.5) normal (0, 0, 1) x (-1, 0, 0)
  line L0 (0, 79) -> (0, 74)
  line L1 (0, 74) -> (117.5, 74)
  line L2 (117.5, 74) -> (117.5, -71.5)
  line L3 (117.5, -71.5) -> (0, -71.5)
  line L4 (0, -71.5) -> (0, -76.5)
  line L5 (0, -76.5) -> (122.5, -76.5)
  line L6 (122.5, -76.5) -> (122.5, 79)
  line L7 (122.5, 79) -> (0, 79)
extrude "Extrude36" add 1 faces at (-108.5, 69.1667, 19.9) along direction (0, 0, 1) blind 2 on bodies 3 bodies 3
extrude "Extrude37" cut 1 faces at (-108.5, 69.1667, 13.9) along direction (0, 0, 1) blind 2 on bodies 3 bodies 3
extrude "Extrude38" add 1 faces at (-108.5, 69.1667, 15.9) along direction (0, 0, -1) blind 0.5 on bodies 3 bodies 3
extrude "Extrude39" cut 1 faces at (-108.5, 69.1667, 21.9) along direction (0, 0, -1) blind 0.5 on bodies 3 bodies 3
sketch "Sketch25" plane through (-117.5, 0, 0) normal (1, 0, 0) x (0, 1, 0)
  line L0 (19.6924, 11.8033) -> (0, 11.8033)
  line L1 (0, 11.8033) -> (0, 26.3373)
  line L2 (0, 26.3373) -> (19.6924, 26.3373)
  line L3 (19.6924, 26.3373) -> (19.6924, 11.8033)
  line L4 (21.6924, 11.8033) -> (21.6924, 26.3373)
  line L5 (21.6924, 26.3373) -> (41.3847, 26.3373)
  line L6 (41.3847, 26.3373) -> (41.3847, 11.8033)
  line L7 (41.3847, 11.8033) -> (21.6924, 11.8033)
  line L8 (71.5, 15.4) -> (51.629, 15.4)
  line L9 (51.629, 15.4) -> (51.629, 21.4)
  line L10 (51.629, 21.4) -> (71.5, 21.4)
  line L11 (71.5, 21.4) -> (71.5, 36.5)
  line L12 (71.5, 36.5) -> (-74, 36.5)
  line L13 (-74, 36.5) -> (-74, 18.9)
  line L14 (-74, 18.9) -> (-54.129, 18.9)
  line L15 (-54.129, 18.9) -> (-54.129, 12.9)
  line L16 (-54.129, 12.9) -> (-74, 12.9)
  line L17 (-74, 12.9) -> (-74, 5)
  line L18 (-74, 5) -> (71.5, 5)
  line L19 (71.5, 5) -> (71.5, 15.4)
  line L20 (51.629, 21.4) -> (43.629, 21.4)
  line L21 (41.3847, 26.3373) -> (43.629, 26.3373)
  line L22 (43.629, 26.3373) -> (43.629, 21.4)
  line L23 (43.629, 21.4) -> (41.3847, 21.4)
  line L24 (41.3847, 21.4) -> (41.3847, 26.3373)
  line L25 (41.3847, 11.8033) -> (43.629, 11.8033)
  line L26 (43.629, 11.8033) -> (43.629, 21.4)
  line L27 (43.629, 21.4) -> (41.3847, 21.4)
  line L28 (41.3847, 21.4) -> (41.3847, 11.8033)
  line L29 (0, 26.3373) -> (4, 26.3373)
  line L30 (4, 26.3373) -> (4, 11.8033)
  line L31 (4, 11.8033) -> (0, 11.8033)
  line L32 (0, 11.8033) -> (0, 26.3373)
  dimension "d147" = 8
  dimension "d148" = 4
  constraint horizontal L20
  constraint coincident L9.end L10.start
  constraint horizontal L21
  constraint vertical L22
  constraint horizontal L23
  constraint vertical L24
  constraint coincident L5.end L6.start
  constraint horizontal L25
  constraint vertical L26
  constraint horizontal L27
  constraint vertical L28
  constraint coincident L6.end L7.start
  constraint horizontal L29
  constraint vertical L30
  constraint horizontal L31
  constraint vertical L32
  constraint coincident L1.end L2.start
  measures "d147" distance of L9.end L20.end
  measures "d148" distance of L1.end L29.end
extrude "Extrude40" cut sketch "Sketch25" against normal blind 5 contours L6 L23 L25 L26 L27 L28 | L6 L21 L22 L23 L24 L27 bodies 3
extrude "Extrude41" add sketch "Sketch25" against normal up to surface (5 mm away) contours L0 L1 L2 L29 L30 L31 L32 bodies 3
extrude "Extrude42" add 1 faces at (-119.1667, 21.6924, 16.648) along direction (0, 1, 0) blind 5 on bodies 3 bodies 3
extrude "Extrude43" cut 1 faces at (-120.8333, 19.6924, 16.648) along direction (0, 1, 0) blind 5 on bodies 3 bodies 3
extrude "Extrude44" add 1 faces at (-120.8333, 24.6924, 16.648) along direction (0, -1, 0) blind 0.5 on bodies 3 bodies 3
extrude "Extrude45" cut 1 faces at (-119.1667, 26.6924, 16.648) along direction (0, -1, 0) blind 0.5 on bodies 3 bodies 3
extrude "Extrude46" cut 1 faces at (-119.1667, 26.1924, 16.648) along direction (0, -1, 0) blind 5 on bodies 3 bodies 3
extrude "Extrude47" cut 1 faces at (85, 73.1667, 22.6667) along direction (1, 0, 0) blind 5.5 on bodies 1 bodies 1
extrude "Extrude48" add 1 faces at (30, 74.8333, 17.3333) along direction (1, 0, 0) blind 5.5 on bodies 1 bodies 1
extrude "Extrude49" cut 1 faces at (90.5, 73.1667, 22.6667) along direction (1, 0, 0) blind 4 on bodies 1 bodies 1
extrude "Extrude50" add 1 faces at (35.5, 74.8333, 17.3333) along direction (1, 0, 0) blind 2 on bodies 1 bodies 1
sketch "Sketch26" plane through (0, 0, 36.5) normal (0, 0, 1) x (-1, 0, 0)
  line L0 (0, 74) -> (0, 79)
  line L1 (0, 79) -> (-122.5, 79)
  line L2 (-122.5, 79) -> (-122.5, -76.5)
  line L3 (-122.5, -76.5) -> (0, -76.5)
  line L4 (0, -76.5) -> (0, -71.5)
  line L5 (0, -71.5) -> (-117.5, -71.5)
  line L6 (-117.5, -71.5) -> (-117.5, 74)
  line L7 (-117.5, 74) -> (0, 74)
  line L8 (-122.5, 79) -> (0, 79)
  line L9 (0, 79) -> (0, -76.5)
  line L10 (0, -76.5) -> (-122.5, -76.5)
  line L11 (-122.5, -76.5) -> (-122.5, 79)
  line L12 (-117.5, 74) -> (0, 74)
  line L13 (0, 74) -> (0, -71.5)
  line L14 (0, -71.5) -> (-117.5, -71.5)
  line L15 (-117.5, -71.5) -> (-117.5, 74)
  constraint horizontal L8
  constraint vertical L9
  constraint horizontal L10
  constraint vertical L11
  constraint coincident L3.end L4.start
  constraint coincident L1.end L2.start
  constraint horizontal L12
  constraint vertical L13
  constraint horizontal L14
  constraint vertical L15
  constraint coincident L4.end L5.start
  constraint coincident L6.end L7.start
extrude "Extrude51" add sketch "Sketch26" along normal blind 8.5 separate body makes body 4
extrude "Extrude52" add 3 faces at (0, 74.8333, 39.3333) (0, -25.5, 39.3333) (0, -75.6667, 39.3333) along direction (-1, 0, 0) up to surface end surface through (-122.5, 24.6924, 11.8033) normal (-1, 0, 0) offset 0 on bodies 4 bodies 4
ref_plane "WorkPlane5" through (-117.5, 0, 0) normal (1, 0, 0) x (0, 1, 0)
sketch "Sketch27" plane through (-117.5, 0, 0) normal (1, 0, 0) x (0, 1, 0)
sketch "Sketch28" plane through (0, 0, 36.5) normal (0, 0, -1) x (1, 0, 0)
  line L0 (-122.5, -76.5) -> (122.5, -76.5)
  line L1 (122.5, -76.5) -> (122.5, 79)
  line L2 (122.5, 79) -> (-122.5, 79)
  line L3 (-122.5, 79) -> (-122.5, -76.5)
sketch "Sketch29" plane through (0, 0, 36.5) normal (0, 0, -1) x (1, 0, 0)
  line L0 (-122.5, -76.5) -> (122.5, -76.5)
  line L1 (122.5, -76.5) -> (122.5, 79)
  line L2 (122.5, 79) -> (-122.5, 79)
  line L3 (-122.5, 79) -> (-122.5, -76.5)
extrude "Extrude53" add sketch "Sketch26" against normal blind 8 contours L5 L6 L7 L9 L12 L13 L14 L15 bodies 4
mirror "Mirror7" about plane through (0, -1.25, 18.25) normal (-1, 0, 0) of 5 faces at (117.5, 23, 33.8333) (78.3333, -25.5, 28.5) (39.1667, 71.5, 31.1667) (78.3333, -74, 31.1667) (0, -25.5, 33.8333) on bodies 4
sketch "Sketch30" plane through (0, 71.5, 0) normal (0, -1, 0) x (1, 0, 0)
  line L0 (-97.5, 21.4) -> (-97.5, 15.4)
  line L1 (-97.5, 15.4) -> (-117.5, 15.4)
  line L2 (-117.5, 15.4) -> (-117.5, 5)
  line L3 (-117.5, 5) -> (0, 5)
  line L4 (0, 5) -> (0, 36.5)
  line L5 (0, 36.5) -> (-117.5, 36.5)
  line L6 (-117.5, 36.5) -> (-117.5, 21.4)
  line L7 (-117.5, 21.4) -> (-97.5, 21.4)
sketch "Sketch31" plane through (-117.5, 0, 0) normal (1, 0, 0) x (0, 1, 0)
  line L0 (43.629, 11.8033) -> (4, 11.8033)
  line L1 (4, 11.8033) -> (4, 26.3373)
  line L2 (4, 26.3373) -> (43.629, 26.3373)
  line L3 (43.629, 26.3373) -> (43.629, 11.8033)
  line L4 (71.5, 15.4) -> (51.629, 15.4)
  line L5 (51.629, 15.4) -> (51.629, 21.4)
  line L6 (51.629, 21.4) -> (71.5, 21.4)
  line L7 (71.5, 21.4) -> (71.5, 36.5)
  line L8 (71.5, 36.5) -> (-74, 36.5)
  line L9 (-74, 36.5) -> (-74, 18.9)
  line L10 (-74, 18.9) -> (-54.129, 18.9)
  line L11 (-54.129, 18.9) -> (-54.129, 12.9)
  line L12 (-54.129, 12.9) -> (-74, 12.9)
  line L13 (-74, 12.9) -> (-74, 5)
  line L14 (-74, 5) -> (71.5, 5)
  line L15 (71.5, 5) -> (71.5, 15.4)
  line L16 (-74, 36.5) -> (71.5, 36.5)
  line L17 (71.5, 36.5) -> (71.5, 5)
  line L18 (71.5, 5) -> (-74, 5)
  line L19 (-74, 5) -> (-74, 36.5)
  line L20 (0, 0) -> (0, 36.5)
  line L21 (25, 27.5) -> (-25, 27.5)
  line L22 (-25, 27.5) -> (-25, 45.5)
  line L23 (-25, 45.5) -> (25, 45.5)
  line L24 (25, 45.5) -> (25, 27.5)
  line L25 (25, 27.5) -> (-25, 45.5) construction
  line L26 (-25, 27.5) -> (25, 45.5) construction
  point P0 (0, 36.5)
  dimension "d180" = 50
  dimension "d181" = 18
  constraint horizontal L16
  constraint vertical L17
  constraint horizontal L18
  constraint vertical L19
  constraint coincident L14.end L15.start
  constraint coincident L8.end L9.start
  constraint coincident L20.start origin
  constraint coincident L16 P0
  constraint perpendicular L16 L20
  constraint horizontal L21
  constraint perpendicular L21 L22
  constraint parallel L21 L23
  constraint parallel L22 L24
  constraint coincident L25 P0
  constraint coincident L26 P0
  constraint coincident P0 L20.end
  measures "d180" distance of L22.end L23.end
  measures "d181" distance of L21.end L22.end
sketch "Sketch33" plane through (-117.5, 0, 0) normal (1, 0, 0) x (0, 1, 0)
  line L0 (43.629, 11.8033) -> (4, 11.8033)
  line L1 (4, 11.8033) -> (4, 26.3373)
  line L2 (4, 26.3373) -> (43.629, 26.3373)
  line L3 (43.629, 26.3373) -> (43.629, 11.8033)
  line L4 (71.5, 15.4) -> (51.629, 15.4)
  line L5 (51.629, 15.4) -> (51.629, 21.4)
  line L6 (51.629, 21.4) -> (71.5, 21.4)
  line L7 (71.5, 21.4) -> (71.5, 36.5)
  line L8 (71.5, 36.5) -> (-74, 36.5)
  line L9 (-74, 36.5) -> (-74, 18.9)
  line L10 (-74, 18.9) -> (-54.129, 18.9)
  line L11 (-54.129, 18.9) -> (-54.129, 12.9)
  line L12 (-54.129, 12.9) -> (-74, 12.9)
  line L13 (-74, 12.9) -> (-74, 5)
  line L14 (-74, 5) -> (71.5, 5)
  line L15 (71.5, 5) -> (71.5, 15.4)
  line L16 (-74, 36.5) -> (71.5, 36.5)
  line L17 (71.5, 36.5) -> (71.5, 28.5)
  line L18 (71.5, 28.5) -> (-74, 28.5)
  line L19 (-74, 28.5) -> (-74, 36.5)
  line L20 (0, 0) -> (0, 36.5)
  line L21 (-74, 36.5) -> (71.5, 36.5)
  line L22 (71.5, 36.5) -> (71.5, 28.5)
  line L23 (71.5, 28.5) -> (-74, 28.5)
  line L24 (-74, 28.5) -> (-74, 36.5)
  line L25 (-74, 32.5) -> (0, 32.5)
  line L26 (22.5, 36.5) -> (-22.5, 36.5)
  line L27 (-22.5, 36.5) -> (-22.5, 28.5)
  line L28 (-22.5, 28.5) -> (22.5, 28.5)
  line L29 (22.5, 28.5) -> (22.5, 36.5)
  line L30 (22.5, 36.5) -> (-22.5, 28.5) construction
  line L31 (-22.5, 36.5) -> (22.5, 28.5) construction
  point P0 (0, 32.5)
  dimension "d188" = 45
  dimension "d189" = 8
  constraint coincident L20.start origin
  constraint coincident L8 L20.end
  constraint perpendicular L8 L20
  constraint horizontal L21
  constraint vertical L22
  constraint horizontal L23
  constraint vertical L24
  constraint coincident L17.end L18.start
  constraint coincident L8.end L9.start
  constraint midpoint L24 L25.start
  constraint coincident L20 P0
  constraint perpendicular L20 L25
  constraint horizontal L26
  constraint perpendicular L26 L27
  constraint parallel L26 L28
  constraint parallel L27 L29
  constraint coincident L30 P0
  constraint coincident L31 P0
  constraint coincident P0 L25.end
  measures "d188" distance of L27.end L28.end
  measures "d189" distance of L26.end L27.end
extrude "Extrude56" add sketch "Sketch33" along normal blind 10 draft -45 contours L8 L16 L18 L20 L21 L23 L26 L28 L29 | L18 L20 L23 L25 L27 L28 | L8 L16 L20 L21 L25 L26 L27 bodies 3
ref_plane "WorkPlane6" through (0, -1.25, 18.25) normal (1, 0, 0) x (0, 1, 0)
mirror "Mirror9" about plane through (0, -1.25, 18.25) normal (1, 0, 0) of "Extrude56" makes body 5
extrude "Extrude57" add 1 faces at (117.5, -7.5, 32.5) along direction (1, 0, 0) blind 5 on bodies 5 bodies 1 3 5
sketch "Sketch34" plane through (117.5, 0, 0) normal (1, 0, 0) x (0, 1, 0)
  line L0 (71.5, 36.5) -> (-74, 36.5)
  line L1 (-74, 36.5) -> (-74, 28.5)
  line L2 (-74, 28.5) -> (71.5, 28.5)
  line L3 (71.5, 28.5) -> (71.5, 36.5)
  line L4 (-22.5, 36.5) -> (-22.5, 28.5)
  line L5 (-22.5, 28.5) -> (22.5, 28.5)
  line L6 (22.5, 28.5) -> (22.5, 36.5)
  line L7 (-22.5, 36.5) -> (22.5, 36.5)
  constraint coincident L4.start L7.start
  constraint coincident L6.end L7.end
extrude "Extrude58" cut sketch "Sketch34" against normal blind 10 draft -45 contours L0 L2 L4 L5 L6 L7 bodies 4
mirror "Mirror10" about plane through (0, -1.25, 18.25) normal (1, 0, 0) of "Extrude58"